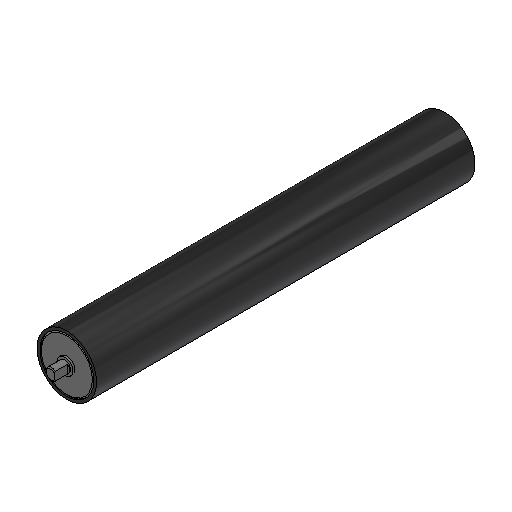
# Autodesk Inventor part: FREE ROLLER
Saved by Autodesk Inventor 2022.5 (Build 265521000, 521)
## iProperties
Created: 2023-04-11
Part Number: FREE ROLLER
Material: SS400
Description: 3
Document SubType Name: Modeling
Designer: 박성규
Density: 7.85 g/cm^3
Appearance: 도금 백색 아연
DETAIL: Coveryor Assembly
M/C TITLE: CJ 제일제당 협동로봇 포장시스탬 PILOT 장비
MAKER: EUNHYUN
PARTS NAME: Bracket
SPECIFICATION: TA20221101-CV200000-015
DocNumber: 221118_Standard_v1
Folder: .\
VDS_Category: 엔지니어링
Detail Description: Purchased products
Title: FR570-400-12-JD-ZN-NR630A
Author: 박성규
Revision Number: B
Autodesk Inventor part; units mm, degrees
ref_plane "YZ Plane" through (0, 0, 0) normal (1, 0, 0) x (0, 1, 0)
ref_plane "XZ Plane" through (0, 0, 0) normal (0, 1, 0) x (-1, 0, 0)
ref_plane "XY Plane" through (0, 0, 0) normal (0, 0, 1) x (1, 0, 0)
sketch "스케치9" plane through (0, 0, 0) normal (0, 0, 1) x (1, 0, 0)
  circle A0 centre (0, 0) radius 28.5
  dimension "d40" = 57
  constraints: 1 centre point, 1 coincident
  measures "d40" diameter of A0
extrude "돌출4" add sketch "스케치9" along normal mid plane 400
sketch "스케치10" plane through (0, 0, 200) normal (0, 0, 1) x (1, 0, 0)
  circle A0 centre (0, 0) radius 28.5 construction
  circle A1 centre (0, 0) radius 24.5
  dimension "d43" = 4
  constraints: 1 centre point
  measures "d43" radial gap between concentric circles of A0 A1
extrude "돌출5" cut sketch "스케치10" against normal through all
sketch "스케치11" plane through (0, 0, 200) normal (0, 0, 1) x (1, 0, 0)
  circle A0 centre (0, 0) radius 28.5 construction
  circle A1 centre (0, 0) radius 28.5
  constraints: 1 centre point, 1 coincident, 1 concentric
extrude "돌출6" add sketch "스케치11" against normal blind 1.5
sketch "스케치12" plane through (0, 0, -200) normal (0, 0, -1) x (-1, 0, 0)
  circle A0 centre (0, 0) radius 28.5 construction
  circle A1 centre (0, 0) radius 28.5
  constraints: 1 centre point, 1 coincident
extrude "돌출7" add sketch "스케치12" against normal blind 1.5
chamfer "모따기1" distance 1.5 angle 45 3 edges at (0, -28.5, -200) (0, 28.5, -200) (-28.5, 0, 200)
sketch "스케치13" plane through (0, 0, 200) normal (0, 0, 1) x (1, 0, 0)
  circle A0 centre (0, 0) radius 27 construction
  circle A1 centre (0, 0) radius 8.5
  dimension "d53" = 17
  constraints: 1 centre point, 1 coincident
  measures "d53" diameter of A1
extrude "돌출8" add sketch "스케치13" along normal blind 2
sketch "스케치14" plane through (0, 0, 202) normal (0, 0, 1) x (1, 0, 0)
  circle A0 centre (0, 0) radius 8.5 construction
  circle A1 centre (0, 0) radius 6
  dimension "d56" = 12
  constraints: 1 centre point, 1 coincident
  measures "d56" diameter of A1
extrude "돌출9" add sketch "스케치14" along normal blind 15
sketch "스케치15" plane through (0, 0, 217) normal (0, 0, 1) x (1, 0, 0)
  circle A0 centre (0, 0) radius 6 construction
  line L0 (39, 16) -> (4, 16)
  line L1 (4, 16) -> (4, -15)
  line L2 (4, -15) -> (39, -15)
  line L3 (39, -15) -> (39, 16)
  dimension "d59" = 4
  constraints: 8 end point, 2 parallel, 1 horizontal, 1 perpendicular
  measures "d59" distance from line of L1 A0.centre
extrude "돌출10" cut sketch "스케치15" against normal blind 14
chamfer "모따기2" distance 1 angle 45 1 edges at (-6, 0, 217)
mirror "미러1" about plane through (0, 0, 0) normal (0, 0, 1) of "돌출8", "돌출9", "돌출10", "모따기2"
sketch "스케치16" plane through (0, 0, 0) normal (0, 0, 1) x (1, 0, 0)
  circle A0 centre (0, 0) radius 6 construction
  circle A1 centre (0, 0) radius 31.5
  circle A2 centre (0, 0) radius 28.5 projected
  dimension "d65" = 63
  constraints: 1 centre point, 1 coincident
  measures "d65" diameter of A1
extrude "돌출11" add sketch "스케치16" along normal mid plane 400 separate body
